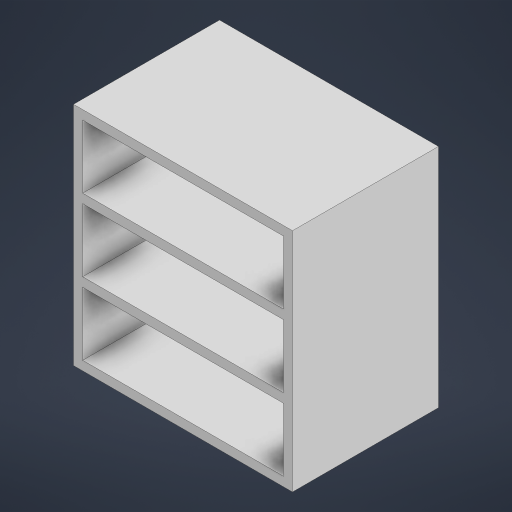
# Autodesk Inventor part: Pensile
Saved by Autodesk Inventor 2024.2 (Build 282272000, 272)
## iProperties
Created: 2025-08-23
Part Number: Pensile
Material: Generic
Document SubType Name: Modeling
Designer: Luca
Density: 1 g/cm^3
Appearance: Default
Author: Luca
Autodesk Inventor part; units mm, degrees
ref_plane "YZ Plane" through (0, 0, 0) normal (1, 0, 0) x (0, 1, 0)
ref_plane "XZ Plane" through (0, 0, 0) normal (0, 1, 0) x (-1, 0, 0)
ref_plane "XY Plane" through (0, 0, 0) normal (0, 0, 1) x (1, 0, 0)
sketch "Sketch1" plane through (0, 0, 0) normal (0, 0, 1) x (1, 0, 0)
  line L0 (-300, 620) -> (300, 620)
  line L1 (300, 620) -> (300, 0)
  line L2 (300, 0) -> (-300, 0)
  line L3 (-300, 0) -> (-300, 620)
  point P0 (0, 0)
  point P1 (0, 0)
  dimension "d0" = 600
  dimension "d1" = 620
  constraints: 8 end point, 2 parallel, 1 coincident, 1 horizontal, 1 midpoint, 1 perpendicular
  measures "d0" distance of L1.end L2.end
  measures "d1" distance of L0.end L1.end
extrude "Extrusion1" add sketch "Sketch1" along normal blind 400
sketch "Sketch2" plane through (0, 0, 400) normal (0, 0, 1) x (1, 0, 0)
  line L0 (-300, 0) -> (300, 0) projected
  line L1 (300, 0) -> (300, 620) projected
  line L2 (300, 620) -> (-300, 620) projected
  line L3 (-300, 620) -> (-300, 0) projected
  line L4 (-275, 595) -> (275, 595)
  line L5 (275, 595) -> (275, 421.6667)
  line L6 (275, 421.6667) -> (-275, 421.6667)
  line L7 (-275, 421.6667) -> (-275, 595)
  line L8 (275, 396.6667) -> (-275, 396.6667)
  line L9 (-275, 396.6667) -> (-275, 223.3333)
  line L10 (-275, 223.3333) -> (275, 223.3333)
  line L11 (275, 223.3333) -> (275, 396.6667)
  line L12 (-275, 198.3333) -> (275, 198.3333)
  line L13 (275, 198.3333) -> (275, 25)
  line L14 (275, 25) -> (-275, 25)
  line L15 (-275, 25) -> (-275, 198.3333)
  line L16 (-275, 421.6667) -> (-275, 396.6667) construction
  line L17 (-275, 223.3333) -> (-275, 198.3333) construction
  line L18 (-275, 595) -> (-300, 620) construction
  line L19 (275, 595) -> (300, 620) construction
  line L20 (-275, 25) -> (-300, 0) construction
  point P0 (0, 0)
  dimension "d4" = 25
  dimension "d5" = 25
  constraints: 34 end point, 12 equal length, 5 perpendicular, 5 point on line, 3 horizontal, 1 vertical
  measures "d4" distance between parallel lines of L8 L6
  measures "d5" distance between parallel lines of L3 L16
extrude "Extrusion2" cut sketch "Sketch2" against normal blind 375 contours L4 L5 L6 L7 | L11 L10 L9 L8 | L12 L13 L14 L15
equation "\"d5\" = d4"
equation "\"d6\" = d2 - d4"
equation "\"d2\" = 400"
body "Solid1"
